Autodesk Fusion 360 part; units mm, degrees
(part 2 of 2)
sketch "Skizze3" plane through (-27, 0, 0) normal (1, 0, 0) x (0, 1, 0)
  line L0 (39, -5) -> (33, -5)
  line L1 (33, -5) -> (33, -3.5)
  line L2 (33, -3.5) -> (39, -3.5)
  line L3 (39, -3.5) -> (39, -5)
  line L4 (12, -3.5) -> (12, -5)
  line L5 (12, -5) -> (6, -5)
  line L6 (6, -5) -> (6, -3.5)
  line L7 (6, -3.5) -> (12, -3.5)
  line L8 (33, -16.5) -> (33, -15)
  line L9 (33, -15) -> (39, -15)
  line L10 (39, -15) -> (39, -16.5)
  line L11 (39, -16.5) -> (33, -16.5)
  line L12 (12, -16.5) -> (6, -16.5)
  line L13 (6, -16.5) -> (6, -15)
  line L14 (6, -15) -> (12, -15)
  line L15 (12, -15) -> (12, -16.5)
  line L16 (0, 0) -> (0, -21)
  line L17 (0, -21) -> (45, -21)
  line L18 (45, -21) -> (45, 0)
  line L19 (0, -21) -> (45, -21)
  line L20 (39, -3.5) -> (33, -3.5)
  line L21 (39, -5) -> (39, -3.5)
  line L22 (33, -5) -> (39, -5)
  line L23 (33, -3.5) -> (33, -5)
  line L24 (6, -3.5) -> (6, -5)
  line L25 (12, -3.5) -> (6, -3.5)
  line L26 (12, -5) -> (12, -3.5)
  line L27 (6, -5) -> (12, -5)
  line L28 (39, -16.5) -> (39, -15)
  line L29 (33, -16.5) -> (39, -16.5)
  line L30 (33, -15) -> (33, -16.5)
  line L31 (39, -15) -> (33, -15)
  line L32 (12, -15) -> (6, -15)
  line L33 (12, -16.5) -> (12, -15)
  line L34 (6, -16.5) -> (12, -16.5)
  line L35 (6, -15) -> (6, -16.5)
  line L36 (0, -21) -> (0, 1)
  line L37 (45, -21) -> (45, 1)
  line L38 (0, -20) -> (45, -20)
  line L39 (45, 0) -> (0, 0)
  line L40 (45, 1) -> (0, 1)
  dimension "d85" = 1
  constraint coincident L36 L38.start
  constraint coincident L37 L38.end
  constraint perpendicular L37 L38
  measures "d85" distance of L17 L38
extrude "Extrusion5" add sketch "Skizze3" along normal up to surface (62 mm away) contours L16 L17 L18 L19 L36 L37 L38
sketch "Skizze4" plane through (0, 0, 0) normal (0, 0, -1) x (1, 0, 0)
  line L0 (-27, -45) -> (-10, -45)
  line L1 (35, -45) -> (35, 0)
  line L2 (35, 0) -> (-10, 0)
  circle A0 centre (25, -6) radius 2
  circle A1 centre (25, -39) radius 2
  line L3 (35, 0) -> (35, -45)
  line L4 (-27, 0) -> (-27, -45)
  line L5 (-28, -45) -> (-28, 0)
  line L6 (-10, -45) -> (35, -45)
  line L7 (-10, 0) -> (-27, 0)
  line L8 (-10, 0) -> (35, 0)
  line L9 (-27, -45) -> (-28, -45)
  circle A2 centre (11, -38.5) radius 1.5
  circle A3 centre (-21, -6.5) radius 1.5
  circle A4 centre (11, -6.5) radius 1.5
  circle A5 centre (-5, -22.5) radius 12.5
  circle A6 centre (-21, -38.5) radius 1.5
  line L10 (35, -45) -> (-10, -45)
  line L11 (-27, 0) -> (-10, 0)
  line L12 (-28, 0) -> (-27, 0)
  line L13 (-10, -45) -> (-27, -45)
extrude "Extrusion6" cut sketch "Skizze4" along normal up to surface (21 mm away) contours A0 | A1

design "Zahnrad"
Autodesk Fusion 360 part; units mm, degrees
sketch "Skizze1" plane through (0, 0, 53) normal (0, 0, 1) x (-1, 0, 0)
  circle A0 centre (0, 0) radius 2.5
  circle A1 centre (0, 0) radius 6.5
  dimension "d70" = 13
  constraint concentric A0 A1
  measures "d70" diameter of A1
extrude "Extrusion1" add sketch "Skizze1" along normal blind 1
sketch "Skizze2" plane through (0, 0, 54) normal (0, 0, 1) x (-1, 0, 0)
  circle A0 centre (0, 0) radius 2.5
  circle A1 centre (0, 0) radius 6.5
  circle A2 centre (0, 0) radius 5.5
  line L0 (0, 0) -> (-6.5, 0) construction
  circle A3 centre (-5.5, 0) radius 0.5
  circle A4 centre (-5.0813, -2.1048) radius 0.5
  circle A5 centre (-3.8891, -3.8891) radius 0.5
  circle A6 centre (-2.1048, -5.0813) radius 0.5
  circle A7 centre (0, -5.5) radius 0.5
  circle A8 centre (2.1048, -5.0813) radius 0.5
  circle A9 centre (3.8891, -3.8891) radius 0.5
  circle A10 centre (5.0813, -2.1048) radius 0.5
  circle A11 centre (5.5, 0) radius 0.5
  circle A12 centre (5.0813, 2.1048) radius 0.5
  circle A13 centre (3.8891, 3.8891) radius 0.5
  circle A14 centre (2.1048, 5.0813) radius 0.5
  circle A15 centre (0, 5.5) radius 0.5
  circle A16 centre (-2.1048, 5.0813) radius 0.5
  circle A17 centre (-3.8891, 3.8891) radius 0.5
  circle A18 centre (-5.0813, 2.1048) radius 0.5
  dimension "d74" = 11
  dimension "d75" = 1
  dimension "d77" = 360
  constraint coincident A0.centre A1.centre
  constraint coincident A1 L0.end
  constraint horizontal L0
  constraint coincident A2 A3.centre
  constraint coincident L0 A3.centre
  measures "d74" diameter of A2
  measures "d75" diameter of A3
extrude "Extrusion2" add sketch "Skizze2" along normal blind 10 contours A2 A3 A4 A5 A6 A7 A8 A9 A10 A11 A12 A13 A14 A15 A16 A17 A18
sketch "Skizze4" plane through (0, 0, 64) normal (0, 0, 1) x (-1, 0, 0)
  circle A0 centre (0, 0) radius 2.5
  arc A1 (-5.4773, -0.4995) -> (-5.2515, -1.6346) centre (0, 0) ccw
  arc A2 (-4.8692, -2.5575) -> (-5.2515, -1.6346) centre (-5.0813, -2.1048) ccw
  arc A3 (-4.8692, -2.5575) -> (-4.2262, -3.5198) centre (0, 0) ccw
  arc A4 (-3.5198, -4.2262) -> (-4.2262, -3.5198) centre (-3.8891, -3.8891) ccw
  arc A5 (-3.5198, -4.2262) -> (-2.5575, -4.8692) centre (0, 0) ccw
  arc A6 (-1.6346, -5.2515) -> (-2.5575, -4.8692) centre (-2.1048, -5.0813) ccw
  arc A7 (-1.6346, -5.2515) -> (-0.4995, -5.4773) centre (0, 0) ccw
  arc A8 (0.4995, -5.4773) -> (-0.4995, -5.4773) centre (0, -5.5) ccw
  arc A9 (0.4995, -5.4773) -> (1.6346, -5.2515) centre (0, 0) ccw
  arc A10 (2.5575, -4.8692) -> (1.6346, -5.2515) centre (2.1048, -5.0813) ccw
  arc A11 (2.5575, -4.8692) -> (3.5198, -4.2262) centre (0, 0) ccw
  arc A12 (4.2262, -3.5198) -> (3.5198, -4.2262) centre (3.8891, -3.8891) ccw
  arc A13 (4.2262, -3.5198) -> (4.8692, -2.5575) centre (0, 0) ccw
  arc A14 (5.2515, -1.6346) -> (4.8692, -2.5575) centre (5.0813, -2.1048) ccw
  arc A15 (5.2515, -1.6346) -> (5.4773, -0.4995) centre (0, 0) ccw
  arc A16 (5.4773, 0.4995) -> (5.4773, -0.4995) centre (5.5, 0) ccw
  arc A17 (5.4773, 0.4995) -> (5.2515, 1.6346) centre (0, 0) ccw
  arc A18 (4.8692, 2.5575) -> (5.2515, 1.6346) centre (5.0813, 2.1048) ccw
  arc A19 (4.8692, 2.5575) -> (4.2262, 3.5198) centre (0, 0) ccw
  arc A20 (3.5198, 4.2262) -> (4.2262, 3.5198) centre (3.8891, 3.8891) ccw
  arc A21 (3.5198, 4.2262) -> (2.5575, 4.8692) centre (0, 0) ccw
  arc A22 (1.6346, 5.2515) -> (2.5575, 4.8692) centre (2.1048, 5.0813) ccw
  arc A23 (1.6346, 5.2515) -> (0.4995, 5.4773) centre (0, 0) ccw
  arc A24 (-0.4995, 5.4773) -> (0.4995, 5.4773) centre (0, 5.5) ccw
  arc A25 (-0.4995, 5.4773) -> (-1.6346, 5.2515) centre (0, 0) ccw
  arc A26 (-2.5575, 4.8692) -> (-1.6346, 5.2515) centre (-2.1048, 5.0813) ccw
  arc A27 (-2.5575, 4.8692) -> (-3.5198, 4.2262) centre (0, 0) ccw
  arc A28 (-4.2262, 3.5198) -> (-3.5198, 4.2262) centre (-3.8891, 3.8891) ccw
  arc A29 (-4.2262, 3.5198) -> (-4.8692, 2.5575) centre (0, 0) ccw
  arc A30 (-5.2515, 1.6346) -> (-4.8692, 2.5575) centre (-5.0813, 2.1048) ccw
  arc A31 (-5.2515, 1.6346) -> (-5.4773, 0.4995) centre (0, 0) ccw
  arc A32 (-5.4773, -0.4995) -> (-5.4773, 0.4995) centre (-5.5, 0) ccw
  circle A33 centre (0, 0) radius 2.5
  circle A34 centre (0, 0) radius 6.5
extrude "Extrusion3" add sketch "Skizze4" along normal blind 1 contours A1 A2 A3 A4 A5 A6 A7 A8 A9 A10 A11 A12 A13 A14 A15 A16 A17 A18 A19 A20 A21 A22 A23 A24 A25 A26 A27 A28 A29 A30 A31 A32 | A34

design "Motor"
Autodesk Fusion 360 part; units mm, degrees
sketch "Skizze1" plane through (0, 0, 0) normal (0, 0, 1) x (1, 0, 0)
  line L0 (-21, 21) -> (21, 21)
  line L1 (21, 21) -> (21, -21)
  line L2 (21, -21) -> (-21, -21)
  line L3 (-21, -21) -> (-21, 21)
  dimension "d1" = 21
  dimension "d2" = 42
  dimension "d3" = 42
  dimension "d4" = 21
  constraint horizontal L0
  constraint vertical L1
  constraint horizontal L2
  constraint vertical L3
  measures "d1" distance of origin L0
  measures "d2" distance of L0.end L1.end
  measures "d3" distance of L1 L3
  measures "d4" distance of origin L1
extrude "Extrusion1" add sketch "Skizze1" along normal blind 10 makes body 1
fillet "Abrundung1" radius 3.5 4 edges at (21, -21, 5) (21, 21, 5) (-21, 21, 5) (-21, -21, 5) on bodies 1
sketch "Skizze1 (2)" plane through (0, 0, 10) normal (0, 0, 1) x (-1, 0, 0) in component "Component"
  arc A0 (21, 17.5) -> (17.5, 21) centre (17.5, 17.5) ccw
  line L0 (17.5, 21) -> (-17.5, 21)
  arc A1 (-17.5, 21) -> (-21, 17.5) centre (-17.5, 17.5) ccw
  line L1 (-21, 17.5) -> (-21, -17.5)
  arc A2 (-21, -17.5) -> (-17.5, -21) centre (-17.5, -17.5) ccw
  line L2 (-17.5, -21) -> (17.5, -21)
  arc A3 (17.5, -21) -> (21, -17.5) centre (17.5, -17.5) ccw
  line L3 (21, -17.5) -> (21, 17.5)
  line L4 (14, -21) -> (-14, -21)
  line L5 (-21, -14) -> (-21, 14)
  line L6 (-14, 21) -> (14, 21)
  line L7 (21, 14) -> (21, -14)
  line L8 (14, -21) -> (21, -14)
  line L9 (-14, -21) -> (-21, -14)
  line L10 (-21, 14) -> (-14, 21)
  line L11 (14, 21) -> (21, 14)
  point P0 (21, -21)
  point P1 (-21, -21)
  point P2 (-21, 21)
  point P3 (21, 21)
  dimension "d27" = 42
  dimension "d28" = 42
  dimension "d29" = 21
  dimension "d30" = 21
  dimension "d31" = 7
  dimension "d32" = 7
  dimension "d33" = 7
  dimension "d34" = 7
  dimension "d35" = 7
  dimension "d36" = 7
  dimension "d37" = 7
  dimension "d38" = 7
  constraint horizontal L4
  constraint vertical L5
  constraint horizontal L6
  constraint vertical L7
  constraint coincident P0 L4
  constraint coincident P0 L7
  constraint coincident P1 L4
  constraint coincident P1 L5
  constraint coincident P2 L5
  constraint coincident P2 L6
  constraint coincident P3 L6
  constraint coincident P3 L7
  measures "d27" distance of P0 P1
  measures "d28" distance of P1 P2
  measures "d29" distance of origin L4
  measures "d30" distance of origin L5
  measures "d31" distance of P0 L4.start
  measures "d32" distance of P0 L7.end
  measures "d33" distance of P1 L4.end
  measures "d34" distance of P1 L5.start
  measures "d35" distance of P2 L5.end
  measures "d36" distance of P2 L6.start
  measures "d37" distance of P3 L6.end
  measures "d38" distance of P3 L7.start
extrude "Extrusion1'" add sketch "Skizze1 (2)" along normal blind 17.5 separate body contours L0 L1 L2 L3 L4 L5 L6 L7 L8 L9 L10 L11 makes body 2 in component "Component"
sketch "Skizze4" plane through (0, 0, 10) normal (0, 0, 1) x (-1, 0, 0)
  arc A0 (21, 17.5) -> (17.5, 21) centre (17.5, 17.5) ccw
  line L0 (17.5, 21) -> (-17.5, 21)
  arc A1 (-17.5, 21) -> (-21, 17.5) centre (-17.5, 17.5) ccw
  line L1 (-21, 17.5) -> (-21, -17.5)
  arc A2 (-21, -17.5) -> (-17.5, -21) centre (-17.5, -17.5) ccw
  line L2 (-17.5, -21) -> (17.5, -21)
  arc A3 (17.5, -21) -> (21, -17.5) centre (17.5, -17.5) ccw
  line L3 (21, -17.5) -> (21, 17.5)
  arc A4 (21, 17.5) -> (17.5, 21) centre (17.5, 17.5) ccw
  line L4 (-17.5, 21) -> (17.5, 21)
  line L5 (21, 17.5) -> (21, -17.5)
  arc A5 (17.5, -21) -> (21, -17.5) centre (17.5, -17.5) ccw
  line L6 (17.5, -21) -> (-17.5, -21)
  arc A6 (-21, -17.5) -> (-17.5, -21) centre (-17.5, -17.5) ccw
  line L7 (-21, -17.5) -> (-21, 17.5)
  arc A7 (-17.5, 21) -> (-21, 17.5) centre (-17.5, 17.5) ccw
  line L8 (14, -21) -> (-14, -21)
  line L9 (-14, -21) -> (-21, -14)
  line L10 (-21, -14) -> (-21, 14)
  line L11 (-21, 14) -> (-14, 21)
  line L12 (-14, 21) -> (14, 21)
  line L13 (14, 21) -> (21, 14)
  line L14 (21, 14) -> (21, -14)
  line L15 (14, -21) -> (21, -14)
extrude "Extrusion4" add sketch "Skizze4" along normal blind 2 contours A0 L0 L3 A4 L4 L5 L13 | L2 A3 L3 L5 A5 L6 L15 | L0 A1 L1 L4 L7 A7 L11 | L1 A2 L2 L6 A6 L7 L9 bodies 1
sketch "Skizze5" plane through (0, 0, 27.5) normal (0, 0, 1) x (-1, 0, 0)
  line L0 (14, -21) -> (21, -14)
  line L1 (21, -14) -> (21, 14)
  line L2 (21, 14) -> (14, 21)
  line L3 (14, 21) -> (-14, 21)
  line L4 (-14, 21) -> (-21, 14)
  line L5 (-21, 14) -> (-21, -14)
  line L6 (-21, -14) -> (-14, -21)
  line L7 (-14, -21) -> (14, -21)
  arc A0 (21, 17.5) -> (17.5, 21) centre (17.5, 17.5) ccw
  line L8 (-17.5, 21) -> (17.5, 21)
  line L9 (21, 17.5) -> (21, -17.5)
  arc A1 (17.5, -21) -> (21, -17.5) centre (17.5, -17.5) ccw
  line L10 (17.5, -21) -> (-17.5, -21)
  arc A2 (-21, -17.5) -> (-17.5, -21) centre (-17.5, -17.5) ccw
  line L11 (-21, -17.5) -> (-21, 17.5)
  arc A3 (-17.5, 21) -> (-21, 17.5) centre (-17.5, 17.5) ccw
sketch "Skizze1 (3)" plane through (0, 0, 27.5) normal (0, 0, 1) x (-1, 0, 0) in component "Component'"
  line L0 (14, -21) -> (21, -14)
  line L1 (21, -14) -> (21, 14)
  line L2 (21, 14) -> (14, 21)
  line L3 (14, 21) -> (-14, 21)
  line L4 (-14, 21) -> (-21, 14)
  line L5 (-21, 14) -> (-21, -14)
  line L6 (-21, -14) -> (-14, -21)
  line L7 (-14, -21) -> (14, -21)
  arc A0 (21, 17.5) -> (17.5, 21) centre (17.5, 17.5) ccw
  line L8 (-17.5, 21) -> (17.5, 21)
  line L9 (21, 17.5) -> (21, -17.5)
  arc A1 (17.5, -21) -> (21, -17.5) centre (17.5, -17.5) ccw
  line L10 (17.5, -21) -> (-17.5, -21)
  arc A2 (-21, -17.5) -> (-17.5, -21) centre (-17.5, -17.5) ccw
  line L11 (-21, -17.5) -> (-21, 17.5)
  arc A3 (-17.5, 21) -> (-21, 17.5) centre (-17.5, 17.5) ccw
extrude "Extrusion1''" add sketch "Skizze1 (3)" along normal blind 10 separate body makes body 3 in component "Component'"
extrude "Extrusion2" add sketch "Skizze5" against normal blind 2 contours L0 L9 A1 L10 | L6 L10 A2 L11 | L2 A0 L8 L9 | L4 L8 L11 A3 bodies 3 in component "Component'"
sketch "Skizze6" plane through (0, 0, 37.5) normal (0, 0, 1) x (-1, 0, 0)
  line L0 (17.5, 21) -> (-17.5, 21)
  arc A0 (-17.5, 21) -> (-21, 17.5) centre (-17.5, 17.5) ccw
  line L1 (-21, 17.5) -> (-21, -17.5)
  arc A1 (-21, -17.5) -> (-17.5, -21) centre (-17.5, -17.5) ccw
  line L2 (-17.5, -21) -> (17.5, -21)
  arc A2 (17.5, -21) -> (21, -17.5) centre (17.5, -17.5) ccw
  line L3 (21, -17.5) -> (21, 17.5)
  arc A3 (21, 17.5) -> (17.5, 21) centre (17.5, 17.5) ccw
  circle A4 centre (0, 0) radius 11
  circle A5 centre (0, 0) radius 3.25
  dimension "d51" = 22
  dimension "d52" = 6.5
  constraint coincident A4.centre A5.centre
  measures "d51" diameter of A4
  measures "d52" diameter of A5
extrude "Extrusion3" add sketch "Skizze6" along normal blind 2 contours A4 bodies 3 in component "Component'"
sketch "Skizze1 (4)" plane through (0, 0, 37.5) normal (0, 0, 1) x (-1, 0, 0) in component "Component''"
  circle A0 centre (0, 0) radius 3.25
  circle A1 centre (0, 0) radius 2.5
  dimension "d63" = 5
  constraint coincident A0.centre A1.centre
  measures "d63" diameter of A1
extrude "Extrusion1'''" add sketch "Skizze1 (4)" along normal blind 15.5 separate body contours A1 makes body 4 in component "Component''"
sketch "Skizze1 (5)" plane through (0, 0, 53) normal (0, 0, 1) x (-1, 0, 0) in component "Component'''"
  circle A0 centre (0, 0) radius 2.5
  circle A1 centre (0, 0) radius 6.5
  dimension "d70" = 13
  constraint concentric A0 A1
  measures "d70" diameter of A1
extrude "Extrusion1''''" add sketch "Skizze1 (5)" along normal blind 1 separate body makes body 5 in component "Component'''"
sketch "Skizze2" plane through (0, 0, 54) normal (0, 0, 1) x (-1, 0, 0) in component "Component'''"
  circle A0 centre (0, 0) radius 2.5
  circle A1 centre (0, 0) radius 6.5
  circle A2 centre (0, 0) radius 5.5
  line L0 (0, 0) -> (-6.5, 0) construction
  circle A3 centre (-5.5, 0) radius 0.5
  circle A4 centre (-5.0813, -2.1048) radius 0.5
  circle A5 centre (-3.8891, -3.8891) radius 0.5
  circle A6 centre (-2.1048, -5.0813) radius 0.5
  circle A7 centre (0, -5.5) radius 0.5
  circle A8 centre (2.1048, -5.0813) radius 0.5
  circle A9 centre (3.8891, -3.8891) radius 0.5
  circle A10 centre (5.0813, -2.1048) radius 0.5
  circle A11 centre (5.5, 0) radius 0.5
  circle A12 centre (5.0813, 2.1048) radius 0.5
  circle A13 centre (3.8891, 3.8891) radius 0.5
  circle A14 centre (2.1048, 5.0813) radius 0.5
  circle A15 centre (0, 5.5) radius 0.5
  circle A16 centre (-2.1048, 5.0813) radius 0.5
  circle A17 centre (-3.8891, 3.8891) radius 0.5
  circle A18 centre (-5.0813, 2.1048) radius 0.5
  dimension "d74" = 11
  dimension "d75" = 1
  dimension "d77" = 360
  constraint coincident A0.centre A1.centre
  constraint coincident A1 L0.end
  constraint horizontal L0
  constraint coincident A2 A3.centre
  constraint coincident L0 A3.centre
  measures "d74" diameter of A2
  measures "d75" diameter of A3
extrude "Extrusion2'" add sketch "Skizze2" along normal blind 10 contours A2 A3 A4 A5 A6 A7 A8 A9 A10 A11 A12 A13 A14 A15 A16 A17 A18 bodies 5 in component "Component'''"
sketch "Skizze4 (2)" plane through (0, 0, 64) normal (0, 0, 1) x (-1, 0, 0) in component "Component'''"
  circle A0 centre (0, 0) radius 2.5
  arc A1 (-5.4773, -0.4995) -> (-5.2515, -1.6346) centre (0, 0) ccw
  arc A2 (-4.8692, -2.5575) -> (-5.2515, -1.6346) centre (-5.0813, -2.1048) ccw
  arc A3 (-4.8692, -2.5575) -> (-4.2262, -3.5198) centre (0, 0) ccw
  arc A4 (-3.5198, -4.2262) -> (-4.2262, -3.5198) centre (-3.8891, -3.8891) ccw
  arc A5 (-3.5198, -4.2262) -> (-2.5575, -4.8692) centre (0, 0) ccw
  arc A6 (-1.6346, -5.2515) -> (-2.5575, -4.8692) centre (-2.1048, -5.0813) ccw
  arc A7 (-1.6346, -5.2515) -> (-0.4995, -5.4773) centre (0, 0) ccw
  arc A8 (0.4995, -5.4773) -> (-0.4995, -5.4773) centre (0, -5.5) ccw
  arc A9 (0.4995, -5.4773) -> (1.6346, -5.2515) centre (0, 0) ccw
  arc A10 (2.5575, -4.8692) -> (1.6346, -5.2515) centre (2.1048, -5.0813) ccw
  arc A11 (2.5575, -4.8692) -> (3.5198, -4.2262) centre (0, 0) ccw
  arc A12 (4.2262, -3.5198) -> (3.5198, -4.2262) centre (3.8891, -3.8891) ccw
  arc A13 (4.2262, -3.5198) -> (4.8692, -2.5575) centre (0, 0) ccw
  arc A14 (5.2515, -1.6346) -> (4.8692, -2.5575) centre (5.0813, -2.1048) ccw
  arc A15 (5.2515, -1.6346) -> (5.4773, -0.4995) centre (0, 0) ccw
  arc A16 (5.4773, 0.4995) -> (5.4773, -0.4995) centre (5.5, 0) ccw
  arc A17 (5.4773, 0.4995) -> (5.2515, 1.6346) centre (0, 0) ccw
  arc A18 (4.8692, 2.5575) -> (5.2515, 1.6346) centre (5.0813, 2.1048) ccw
  arc A19 (4.8692, 2.5575) -> (4.2262, 3.5198) centre (0, 0) ccw
  arc A20 (3.5198, 4.2262) -> (4.2262, 3.5198) centre (3.8891, 3.8891) ccw
  arc A21 (3.5198, 4.2262) -> (2.5575, 4.8692) centre (0, 0) ccw
  arc A22 (1.6346, 5.2515) -> (2.5575, 4.8692) centre (2.1048, 5.0813) ccw
  arc A23 (1.6346, 5.2515) -> (0.4995, 5.4773) centre (0, 0) ccw
  arc A24 (-0.4995, 5.4773) -> (0.4995, 5.4773) centre (0, 5.5) ccw
  arc A25 (-0.4995, 5.4773) -> (-1.6346, 5.2515) centre (0, 0) ccw
  arc A26 (-2.5575, 4.8692) -> (-1.6346, 5.2515) centre (-2.1048, 5.0813) ccw
  arc A27 (-2.5575, 4.8692) -> (-3.5198, 4.2262) centre (0, 0) ccw
  arc A28 (-4.2262, 3.5198) -> (-3.5198, 4.2262) centre (-3.8891, 3.8891) ccw
  arc A29 (-4.2262, 3.5198) -> (-4.8692, 2.5575) centre (0, 0) ccw
  arc A30 (-5.2515, 1.6346) -> (-4.8692, 2.5575) centre (-5.0813, 2.1048) ccw
  arc A31 (-5.2515, 1.6346) -> (-5.4773, 0.4995) centre (0, 0) ccw
  arc A32 (-5.4773, -0.4995) -> (-5.4773, 0.4995) centre (-5.5, 0) ccw
  circle A33 centre (0, 0) radius 2.5
  circle A34 centre (0, 0) radius 6.5
extrude "Extrusion3'" add sketch "Skizze4 (2)" along normal blind 1 contours A1 A2 A3 A4 A5 A6 A7 A8 A9 A10 A11 A12 A13 A14 A15 A16 A17 A18 A19 A20 A21 A22 A23 A24 A25 A26 A27 A28 A29 A30 A31 A32 | A34 bodies 5 in component "Component'''"
sketch "Skizze7" plane through (0, 0, 37.5) normal (0, 0, 1) x (-1, 0, 0)
  line L0 (17.5, 21) -> (-17.5, 21)
  arc A0 (-17.5, 21) -> (-21, 17.5) centre (-17.5, 17.5) ccw
  line L1 (-21, 17.5) -> (-21, -17.5)
  arc A1 (-21, -17.5) -> (-17.5, -21) centre (-17.5, -17.5) ccw
  line L2 (-17.5, -21) -> (17.5, -21)
  arc A2 (17.5, -21) -> (21, -17.5) centre (17.5, -17.5) ccw
  line L3 (21, -17.5) -> (21, 17.5)
  arc A3 (21, 17.5) -> (17.5, 21) centre (17.5, 17.5) ccw
  circle A4 centre (0, 0) radius 11
  arc A5 (17.5, -21) -> (21, -17.5) centre (17.5, -17.5) ccw
  line L4 (17.5, -21) -> (14, -21)
  line L5 (21, -14) -> (21, -17.5)
  arc A6 (21, 17.5) -> (17.5, 21) centre (17.5, 17.5) ccw
  line L6 (21, 17.5) -> (21, 14)
  line L7 (14, 21) -> (17.5, 21)
  arc A7 (-21, -17.5) -> (-17.5, -21) centre (-17.5, -17.5) ccw
  line L8 (-21, -17.5) -> (-21, -14)
  line L9 (-14, -21) -> (-17.5, -21)
  line L10 (-17.5, 21) -> (-14, 21)
  line L11 (-21, 14) -> (-21, 17.5)
  arc A8 (-17.5, 21) -> (-21, 17.5) centre (-17.5, 17.5) ccw
  line L12 (14, -21) -> (-14, -21)
  line L13 (-21, -14) -> (-21, 14)
  line L14 (-14, 21) -> (14, 21)
  line L15 (21, 14) -> (21, -14)
  line L16 (16, -16) -> (-16, -16) construction
  line L17 (-16, -16) -> (-16, 16) construction
  line L18 (-16, 16) -> (16, 16) construction
  line L19 (16, 16) -> (16, -16) construction
  circle A9 centre (16, -16) radius 1.5
  circle A10 centre (16, 16) radius 1.5
  circle A11 centre (-16, 16) radius 1.5
  circle A12 centre (-16, -16) radius 1.5
  dimension "d86" = 16
  dimension "d87" = 32
  dimension "d88" = 16
  dimension "d89" = 32
  dimension "d90" = 3
  dimension "d91" = 3
  dimension "d92" = 3
  dimension "d93" = 3
  constraint horizontal L16
  constraint vertical L17
  constraint horizontal L18
  constraint vertical L19
  constraint coincident L16.start L19.end
  constraint coincident L18.end L19.start
  constraint coincident L17.end L18.start
  constraint coincident L16.end L17.start
  measures "d86" distance of A4.centre L18
  measures "d87" distance of L16.end L17.end
  measures "d88" distance of A4.centre L17
  measures "d89" distance of L17.end L18.end
  measures "d90" diameter of A9
  measures "d91" diameter of A10
  measures "d92" diameter of A11
  measures "d93" diameter of A12
extrude "Extrusion4'" cut sketch "Skizze7" against normal blind 5 contours A9 | A10 | A11 | A12 bodies 3 in component "Component'"
thread "Gewinde1" "ISO Metric profile 3.0 M3x0.5 6H" major diameter 3.086 minor diameter 2.529 pitch 0.5 angle 60 resizes the face on face at (-14.5075, 16.1494, 34.1667) on face at (-17.4981, -15.9252, 34.1667) on face at (17.4925, 16.1494, 34.1667) on face at (14.5019, -15.9252, 34.1667) on bodies 3 in component "Component'"
chamfer "Fase1" distance 0.2 angle 45 4 edges at (17.1789, 15.5427, 37.5) (-14.8211, 15.5427, 37.5) (17.1789, -16.4573, 37.5) (-14.8211, -16.4573, 37.5) on bodies 3 in component "Component'"
chamfer "Fase1'" distance 0.2 angle 45 1 edges at (2.3308, 0.904, 53) on bodies 4 in component "Component''"
component "Component" placed x (1, 0, 0) y (0, 1, 0) z (0, 0, 1) at (0, 0, 0)
component "Component'" placed x (1, 0, 0) y (0, 1, 0) z (0, 0, 1) at (0, 0, 0)
component "Component''" placed x (1, 0, 0) y (0, 1, 0) z (0, 0, 1) at (0, 0, 0)
component "Component'''" placed x (1, 0, 0) y (0, 1, 0) z (0, 0, 1) at (0, 0, -12)
equation "d32 = d31"
equation "d34 = d33"
equation "d36 = d35"
equation "d38 = d37"
